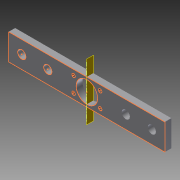
# Autodesk Inventor part: simple_chuck
Saved by Autodesk Inventor 2011 (Build 150239000, 239)
## iProperties
Created: 2012-06-13
Part Number: simple_chuck
Document SubType Name: Modeling
Designer: labuser
Density: 1 g/cm^3
Author: labuser
Autodesk Inventor part; units mm, degrees
ref_plane "YZ Plane" through (0, 0, 0) normal (1, 0, 0) x (0, 1, 0)
ref_plane "XZ Plane" through (0, 0, 0) normal (0, 1, 0) x (-1, 0, 0)
ref_plane "XY Plane" through (0, 0, 0) normal (0, 0, 1) x (1, 0, 0)
sketch "Sketch1" plane through (0, 0, 0) normal (0, 0, 1) x (1, 0, 0)
  circle A0 centre (0, 0) radius 6.477 construction
  circle A1 centre (0, 0) radius 4.75 construction
  circle A2 centre (0, 0) radius 9.525 construction
  line L0 (-38.1, -6.35) -> (38.1, -6.35) construction
  line L1 (38.1, -6.35) -> (38.1, 6.35) construction
  line L2 (38.1, 6.35) -> (-38.1, 6.35) construction
  line L3 (-38.1, 6.35) -> (-38.1, -6.35) construction
  line L4 (-38.1, 6.35) -> (38.1, 6.35)
  line L5 (38.1, 6.35) -> (38.1, -6.35)
  line L6 (38.1, -6.35) -> (-38.1, -6.35)
  line L7 (-38.1, -6.35) -> (-38.1, 6.35)
  dimension "d0" = 12.954
  dimension "d1" = 9.5
  dimension "d2" = 19.05
  dimension "d3" = 76.2
  dimension "d4" = 12.7
  constraints: 16 end point, 4 parallel, 3 centre point, 3 coincident, 2 horizontal, 2 perpendicular
  measures "d0" diameter of A0
  measures "d1" diameter of A1
  measures "d2" diameter of A2
  measures "d3" distance of L2.end L1.end
  measures "d4" distance of L1.end L0.end
extrude "Extrusion1" add sketch "Sketch1" along normal blind 3.175
sketch "Sketch2" plane through (0, 0, 3.175) normal (0, 0, 1) x (1, 0, 0)
  circle A0 centre (0, 0) radius 5.25
  dimension "d7" = 10.5
  constraints: 1 centre point, 1 coincident
  measures "d7" diameter of A0
extrude "Extrusion2" cut sketch "Sketch2" against normal through all
sketch "Sketch4" plane through (0, 0, 3.175) normal (0, 0, 1) x (1, 0, 0)
  circle A0 centre (0, 0) radius 5.25 projected
  circle A1 centre (0, 0) radius 7.5 construction
  arc A2 (6.4952, 3.75) -> (-6.4952, 3.75) centre (0, 0) ccw construction
  line L0 (0, 0) -> (6.4952, 3.75) construction
  line L1 (0, 0) -> (7.5, 0) construction
  line L2 (0, 0) -> (-6.4952, 3.75) construction
  point P0 (6.4952, 3.75)
  dimension "d13" = 15
  dimension "d14" = 30
  dimension "d15" = 120
  constraints: 6 end point, 4 point on circle, 3 coincident, 2 centre point, 1 equal length, 1 horizontal
  measures "d13" diameter of A1
  measures "d14" angle of L1 L0
  measures "d15" angle of L0 L2
hole "Hole1" at (-6.4952, 3.75, 3.175) at (6.4952, 3.75, 3.175) direction (0, 0, -1) diameter 1.7018 end through all
sketch "Sketch5" plane through (0, 0, 3.175) normal (0, 0, 1) x (1, 0, 0)
  circle A0 centre (6.4952, 3.75) radius 0.8509 projected
  circle A1 centre (-6.4952, 3.75) radius 0.8509 projected
  circle A2 centre (0, 0) radius 5.25 projected
  line L0 (38.1, -6.35) -> (-38.1, -6.35) projected
  line L1 (38.1, 6.35) -> (38.1, -6.35) projected
  line L2 (-38.1, 6.35) -> (38.1, 6.35) projected
  line L3 (-38.1, -6.35) -> (-38.1, 6.35) projected
  line L4 (-30.9265, 0) -> (29.6642, 0) construction
  constraints: 2 end point, 1 perpendicular
ref_plane "Work Plane1" through (-30.9265, 0, 3.175) normal (0, -1, 0) x (1, 0, 0)
mirror "Mirror1" about plane through (-30.9265, 0, 3.175) normal (0, -1, 0) of "Hole1"
sketch "Sketch6" plane through (0, 0, 3.175) normal (0, 0, 1) x (1, 0, 0)
  point P0 (-31.75, 0)
  point P1 (-19.05, 0)
hole "Hole2" at (-31.75, 0, 3.175) at (-19.05, 0, 3.175) direction (0, 0, -1) diameter 4 end through all
sketch "Sketch7" plane through (0, 0, 3.175) normal (0, 0, 1) x (1, 0, 0)
  circle A0 centre (-19.05, 0) radius 2 projected
  circle A1 centre (-31.75, 0) radius 2 projected
  circle A2 centre (6.4952, -3.75) radius 0.8509 projected
  circle A3 centre (-6.4952, -3.75) radius 0.8509 projected
  circle A4 centre (6.4952, 3.75) radius 0.8509 projected
  circle A5 centre (-6.4952, 3.75) radius 0.8509 projected
  circle A6 centre (0, 0) radius 5.25 projected
  line L0 (38.1, -6.35) -> (-38.1, -6.35) projected
  line L1 (38.1, 6.35) -> (38.1, -6.35) projected
  line L2 (-38.1, 6.35) -> (38.1, 6.35) projected
  line L3 (-38.1, -6.35) -> (-38.1, 6.35) projected
  line L4 (0, 12.6269) -> (0, -12.6269) construction
  constraints: 2 end point, 1 parallel
ref_plane "Work Plane2" through (0, 12.6269, 3.175) normal (-1, 0, 0) x (0, -1, 0)
mirror "Mirror2" about plane through (0, 12.6269, 3.175) normal (-1, 0, 0) of "Hole2"
body "Solid1"
